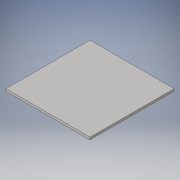
# Autodesk Inventor part: Floor Tile Box O' Doom
Saved by Autodesk Inventor 2016 (Build 200138000, 138)
## iProperties
Created: 2015-09-15
Part Number: Floor Tile Box O' Doom
Material: Generic
Document SubType Name: Modeling
Designer: tbloo
Density: 1 g/cm^3
Appearance: Default
Author: tbloo
Autodesk Inventor part; units mm, degrees
ref_plane "YZ Plane" through (0, 0, 0) normal (1, 0, 0) x (0, 1, 0)
ref_plane "XZ Plane" through (0, 0, 0) normal (0, 1, 0) x (-1, 0, 0)
ref_plane "XY Plane" through (0, 0, 0) normal (0, 0, 1) x (1, 0, 0)
sketch "Sketch1" plane through (0, 0, 0) normal (0, 1, 0) x (-1, 0, 0)
  line L0 (-228.6, -228.6) -> (228.6, -228.6)
  line L1 (228.6, -228.6) -> (228.6, 228.6)
  line L2 (228.6, 228.6) -> (-228.6, 228.6)
  line L3 (-228.6, 228.6) -> (-228.6, -228.6)
  line L4 (-228.6, -228.6) -> (228.6, 228.6) construction
  line L5 (228.6, -228.6) -> (-228.6, 228.6) construction
  point P0 (0, 0)
  dimension "d0" = 457.2
  dimension "d1" = 457.2
  constraints: 12 end point, 2 midpoint, 2 parallel, 1 horizontal, 1 perpendicular
  measures "d0" distance of L2.end L1.end
  measures "d1" distance of L1.end L0.end
extrude "Extrusion1" add sketch "Sketch1" along normal blind 12.7
body "Solid1"
